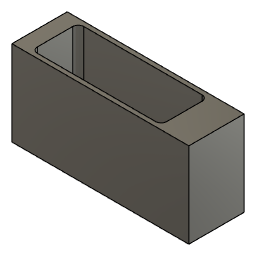
Teste2 (Autodesk Fusion 360 design; units mm, degrees)
Autodesk Fusion 360 part; units mm, degrees
sketch "Esboço1" plane through (0, 0, 0) normal (0, 1, 0) x (1, 0, 0)
  line L0 (0, 0) -> (160, 0)
  line L1 (160, 0) -> (160, -50)
  line L2 (160, -50) -> (0, -50)
  line L3 (0, -50) -> (0, 0)
  dimension "d1" = 160
  dimension "d2" = 50
  constraint horizontal L0
  constraint vertical L1
  constraint horizontal L2
  constraint vertical L3
  constraint coincident L0.start L3.end
  measures "d1" distance of L0.start L0.end
  measures "d2" distance of L0.start L2.end
extrude "Extrusão1" add sketch "Esboço1" along normal blind 77
sketch "Esboço2" plane through (0, 77, 0) normal (0, 1, 0) x (-1, 0, 0)
  line L0 (0, 50) -> (-160, 50)
  line L1 (-160, 50) -> (-160, 0)
  line L2 (-160, 0) -> (0, 0)
  line L3 (0, 0) -> (0, 50)
  line L4 (-131, 46) -> (-14, 46)
  line L5 (-14, 46) -> (-14, 4)
  line L6 (-14, 4) -> (-131, 4)
  line L7 (-131, 4) -> (-131, 46)
  dimension "d5" = 117
  dimension "d6" = 42
  dimension "d7" = 4
  dimension "d8" = 4
  dimension "d9" = 14
  constraint horizontal L4
  constraint vertical L5
  constraint horizontal L6
  constraint vertical L7
  measures "d5" distance of L4.start L4.end
  measures "d6" distance of L4.start L6.end
  measures "d7" distance of L0 L4
  measures "d8" distance of L2 L6
  measures "d9" distance of L3 L5
extrude "Extrusão2" cut sketch "Esboço2" against normal blind 75 contours L4 L5 L6 L7
fillet "Arredondamento1" radius 5 8 edges at (14, 2, 25) (14, 39.5, 4) (14, 39.5, 46) (72.5, 2, 4) (131, 39.5, 4) (131, 2, 25) (72.5, 2, 46) (131, 39.5, 46)
